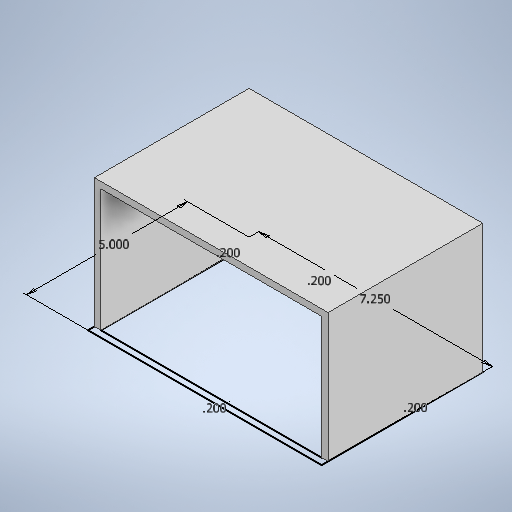
# Autodesk Inventor part: Box_Top
Saved by Autodesk Inventor 2025.1 (Build 291241020, 241B)
## iProperties
Created: 2025-03-03
Part Number: Box_Top
Material: Generic
Document SubType Name: Modeling
Designer: brett
Density: 1 g/cm^3
Appearance: Default
Author: brett
Autodesk Inventor part; units mm, degrees
ref_plane "YZ Plane" through (0, 0, 0) normal (1, 0, 0) x (0, 1, 0)
ref_plane "XZ Plane" through (0, 0, 0) normal (0, 1, 0) x (-1, 0, 0)
ref_plane "XY Plane" through (0, 0, 0) normal (0, 0, 1) x (1, 0, 0)
sketch "Sketch2" plane through (0, 0, 0) normal (0, 1, 0) x (-1, 0, 0)
  line L0 (0, 0) -> (184.15, 0)
  line L1 (184.15, 0) -> (184.15, -127)
  line L2 (184.15, -127) -> (0, -127)
  line L3 (0, -127) -> (0, 0)
  line L4 (179.07, -121.92) -> (5.08, -121.92)
  line L5 (5.08, -121.92) -> (5.08, -5.08)
  line L6 (5.08, -5.08) -> (179.07, -5.08)
  line L7 (179.07, -5.08) -> (179.07, -121.92)
  dimension "d0" = 184.15
  dimension "d1" = 127
  dimension "d2" = 5.08
  dimension "d3" = 5.08
  dimension "d4" = 5.08
  dimension "d5" = 5.08
  constraints: 16 end point, 4 parallel, 2 horizontal, 2 perpendicular
  measures "d0" distance of L1.end L2.end
  measures "d1" distance of L0.end L1.end
  measures "d2" distance between parallel lines of L1 L7
  measures "d3" distance between parallel lines of L3 L5
  measures "d4" distance between parallel lines of L2 L4
  measures "d5" distance between parallel lines of L0 L6
extrude "Extrusion1" add sketch "Sketch2" along normal blind 101.6 contours L0 L1 L2 L3 | L4 L5 L6 L7
extrude "Extrusion2" cut sketch "Sketch2" along normal blind 96.52 contours L4 L5 L6 L7
sketch "Sketch3" plane through (-184.15, 0, 0) normal (0, 0, 1) x (1, 0, 0)
  line L0 (184.15, 0) -> (184.15, 101.6) projected
  line L1 (184.15, 0) -> (0, 0)
  line L2 (0, 0) -> (0, 101.6)
  line L3 (0, 101.6) -> (184.15, 101.6)
  line L4 (184.15, 101.6) -> (184.15, 0)
  dimension "d10" = 184.15
  dimension "d11" = 101.6
  constraints: 8 end point, 2 parallel, 1 horizontal, 1 perpendicular
  measures "d10" distance of L2.end L3.end
  measures "d11" distance of L1.end L2.end
extrude "Extrusion3" cut sketch "Sketch3" against normal up to surface (5.08 mm away)
body "Solid1"
